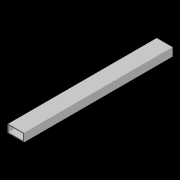
# Autodesk Inventor part: Bolt On Cross Supprot
Saved by Autodesk Inventor 2014 SP1 (Build 180222100, 222)
## iProperties
Created: 2013-11-29
Part Number: Bolt On Cross Supprot
Material: Aluminum 6061
Document SubType Name: Modeling
Designer: Rauhul Varma
Mass: 546.88 g
Surface Area: 1280.01 cm^2
Volume: 201.801 cm^3
Density: 2.71 g/cm^3
Appearance: Aluminum - Flat
Author: Rauhul Varma
Autodesk Inventor part; units mm, degrees
ref_plane "YZ Plane" through (0, 0, 0) normal (1, 0, 0) x (0, 1, 0)
ref_plane "XZ Plane" through (0, 0, 0) normal (0, 1, 0) x (-1, 0, 0)
ref_plane "XY Plane" through (0, 0, 0) normal (0, 0, 1) x (1, 0, 0)
sketch "Sketch1" plane through (0, 0, 0) normal (0, 0, 1) x (1, 0, 0)
  line L0 (0, 0) -> (50.8, 0)
  line L1 (50.8, 0) -> (50.8, 25.4)
  line L2 (50.8, 25.4) -> (0, 25.4)
  line L3 (0, 25.4) -> (0, 0)
  line L4 (3.175, 3.175) -> (47.625, 3.175)
  line L5 (47.625, 3.175) -> (47.625, 22.225)
  line L6 (47.625, 22.225) -> (3.175, 22.225)
  line L7 (3.175, 22.225) -> (3.175, 3.175)
  dimension "d0" = 50.8
  dimension "d1" = 25.4
  dimension "d2" = 3.175
  dimension "d3" = 3.175
  dimension "d4" = 3.175
  dimension "d5" = 3.175
  constraints: 16 end point, 4 parallel, 2 horizontal, 2 perpendicular
  measures "d0" distance of L2.end L1.end
  measures "d1" distance of L1.end L0.end
  measures "d2" distance between parallel lines of L3 L7
  measures "d3" distance between parallel lines of L2 L6
  measures "d4" distance between parallel lines of L0 L4
  measures "d5" distance between parallel lines of L5 L1
extrude "Extrusion1" add sketch "Sketch1" along normal blind 457.2
fillet "Fillet1" radius 3.175 1 edges at (0, 25.4, 228.6)
equation "\"d3\" = d2"
equation "\"d4\" = d2"
equation "\"d5\" = d3"
body "Solid1"
